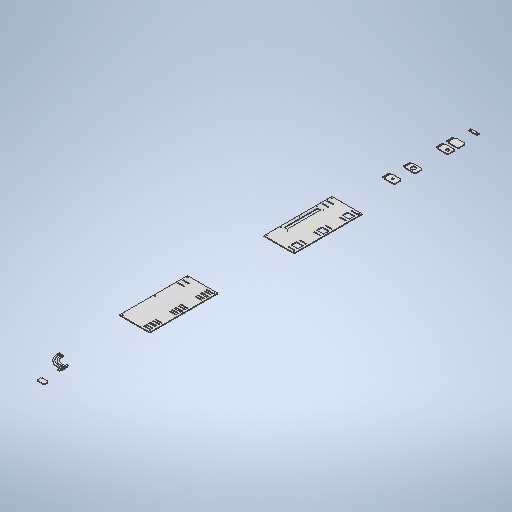
# Autodesk Inventor part: RAW_CHASSIS
Saved by Autodesk Inventor 2025 (Build 290162000, 162)
## iProperties
Created: 2024-11-01
Part Number: RAW_CHASSIS
Material: Generic
Document SubType Name: Modeling
Designer: Student
Density: 1 g/cm^3
Appearance: Default
Author: Student
Autodesk Inventor part; units mm, degrees
ref_plane "YZ Plane" through (0, 0, 0) normal (1, 0, 0) x (0, 1, 0)
ref_plane "XZ Plane" through (0, 0, 0) normal (0, 1, 0) x (-1, 0, 0)
ref_plane "XY Plane" through (0, 0, 0) normal (0, 0, 1) x (1, 0, 0)
sketch "Sketch1" plane through (0, 0, 0) normal (0, 1, 0) x (-1, 0, 0)
  point P0 (0, 0)
sketch "Sketch2" plane through (0, 0, 0) normal (0, 1, 0) x (-1, 0, 0)
  line L0 (-100, 225) -> (100, 225)
  line L1 (100, 225) -> (100, -225)
  line L2 (100, -225) -> (-100, -225)
  line L3 (-100, -225) -> (-100, 225)
  line L4 (-85, -35) -> (-45, -35)
  line L5 (-45, -35) -> (-45, -40)
  line L6 (-45, -40) -> (-85, -40)
  line L7 (-85, -40) -> (-85, -35)
  line L8 (-85, -35) -> (-45, -40) construction
  line L9 (-45, -35) -> (-85, -40) construction
  line L10 (-85, 35) -> (-45, 35)
  line L11 (-45, 35) -> (-45, 40)
  line L12 (-45, 40) -> (-85, 40)
  line L13 (-85, 40) -> (-85, 35)
  line L14 (-87.5, 188) -> (-42.5, 188)
  line L15 (-42.5, 188) -> (-42.5, 152)
  line L16 (-42.5, 152) -> (-87.5, 152)
  line L17 (-87.5, 152) -> (-87.5, 188)
  line L18 (-87.5, 188) -> (-42.5, 152) construction
  line L19 (-42.5, 188) -> (-87.5, 152) construction
  line L20 (-87.5, -188) -> (-42.5, -188)
  line L21 (-42.5, -188) -> (-42.5, -152)
  line L22 (-42.5, -152) -> (-87.5, -152)
  line L23 (-87.5, -152) -> (-87.5, -188)
  line L24 (-87.5, -188) -> (-42.5, -152) construction
  line L25 (-42.5, -188) -> (-87.5, -152) construction
  line L26 (-87.5, 18) -> (-42.5, 18)
  line L27 (-42.5, 18) -> (-42.5, -18)
  line L28 (-42.5, -18) -> (-87.5, -18)
  line L29 (-87.5, -18) -> (-87.5, 18)
  line L30 (-87.5, 18) -> (-42.5, -18) construction
  line L31 (-42.5, 18) -> (-87.5, -18) construction
  line L32 (100, 0) -> (70, 0)
  circle A0 centre (91, 120) radius 3
  circle A1 centre (49, 120) radius 3
  circle A2 centre (91, -120) radius 3
  circle A3 centre (49, -120) radius 3
  line L33 (50, -150) -> (90, -150)
  line L34 (90, -150) -> (90, -155)
  line L35 (90, -155) -> (50, -155)
  line L36 (50, -155) -> (50, -150)
  line L37 (50, -150) -> (90, -155) construction
  line L38 (90, -150) -> (50, -155) construction
  line L39 (50, -182) -> (90, -182)
  line L40 (90, -182) -> (90, -187)
  line L41 (90, -187) -> (50, -187)
  line L42 (50, -187) -> (50, -182)
  line L43 (50, -182) -> (90, -187) construction
  line L44 (90, -182) -> (50, -187) construction
  line L45 (60, 110) -> (80, 110)
  line L46 (80, 110) -> (80, -110)
  line L47 (80, -110) -> (60, -110)
  line L48 (60, -110) -> (60, 110)
  line L49 (60, 110) -> (80, -110) construction
  line L50 (80, 110) -> (60, -110) construction
  line L51 (100, 225) -> (80, 225)
  circle A4 centre (90, 215) radius 3
  circle A5 centre (90, -215) radius 3
  circle A6 centre (90, 0) radius 3
  circle A7 centre (-90, 215) radius 3
  circle A8 centre (-90, -215) radius 3
  circle A9 centre (-94, 0) radius 3
  line L52 (-76.0906, 1157.7188) -> (123.9094, 1157.7188)
  line L53 (123.9094, 1157.7188) -> (123.9094, 707.7188)
  line L54 (123.9094, 707.7188) -> (-76.0906, 707.7188)
  line L55 (-76.0906, 707.7188) -> (-76.0906, 1157.7188)
  line L56 (-61.0906, 1067.7188) -> (-21.0906, 1067.7188)
  line L57 (-21.0906, 1067.7188) -> (-21.0906, 1062.7188)
  line L58 (-21.0906, 1062.7188) -> (-61.0906, 1062.7188)
  line L59 (-61.0906, 1062.7188) -> (-61.0906, 1067.7188)
  line L60 (-61.0906, 1067.7188) -> (-21.0906, 1062.7188) construction
  line L61 (-21.0906, 1067.7188) -> (-61.0906, 1062.7188) construction
  line L62 (-61.0906, 897.7188) -> (-21.0906, 897.7188)
  line L63 (-21.0906, 897.7188) -> (-21.0906, 892.7188)
  line L64 (-21.0906, 892.7188) -> (-61.0906, 892.7188)
  line L65 (-61.0906, 892.7188) -> (-61.0906, 897.7188)
  line L66 (-61.0906, 897.7188) -> (-21.0906, 892.7188) construction
  line L67 (-21.0906, 897.7188) -> (-61.0906, 892.7188) construction
  line L68 (73.9094, 782.7188) -> (113.9094, 782.7188)
  line L69 (113.9094, 782.7188) -> (113.9094, 777.7188)
  line L70 (113.9094, 777.7188) -> (73.9094, 777.7188)
  line L71 (73.9094, 777.7188) -> (73.9094, 782.7188)
  line L72 (73.9094, 782.7188) -> (113.9094, 777.7188) construction
  line L73 (113.9094, 782.7188) -> (73.9094, 777.7188) construction
  line L74 (73.9094, 750.7188) -> (113.9094, 750.7188)
  line L75 (113.9094, 750.7188) -> (113.9094, 745.7188)
  line L76 (113.9094, 745.7188) -> (73.9094, 745.7188)
  line L77 (73.9094, 745.7188) -> (73.9094, 750.7188)
  line L78 (73.9094, 750.7188) -> (113.9094, 745.7188) construction
  line L79 (113.9094, 750.7188) -> (73.9094, 745.7188) construction
  line L80 (123.9094, 1157.7188) -> (103.9094, 1157.7188)
  circle A10 centre (113.9094, 1147.7188) radius 3
  circle A11 centre (113.9094, 717.7188) radius 3
  circle A12 centre (113.9094, 932.7188) radius 3
  circle A13 centre (-66.0906, 1147.7188) radius 3
  circle A14 centre (-66.0906, 717.7188) radius 3
  circle A15 centre (-70.0906, 932.7188) radius 3
  line L81 (-61.0906, 1096.7188) -> (-21.0906, 1096.7188)
  line L82 (-21.0906, 1096.7188) -> (-21.0906, 1108.7188)
  line L83 (-21.0906, 1108.7188) -> (-61.0906, 1108.7188)
  line L84 (-61.0906, 1108.7188) -> (-61.0906, 1096.7188)
  line L85 (-61.0906, 1096.7188) -> (-21.0906, 1108.7188) construction
  line L86 (-21.0906, 1096.7188) -> (-61.0906, 1108.7188) construction
  line L87 (-61.0906, 938.7188) -> (-21.0906, 938.7188)
  line L88 (-21.0906, 938.7188) -> (-21.0906, 926.7188)
  line L89 (-21.0906, 926.7188) -> (-61.0906, 926.7188)
  line L90 (-61.0906, 926.7188) -> (-61.0906, 938.7188)
  line L91 (-61.0906, 938.7188) -> (-21.0906, 926.7188) construction
  line L92 (-21.0906, 938.7188) -> (-61.0906, 926.7188) construction
  line L93 (-61.0906, 768.7188) -> (-21.0906, 768.7188)
  line L94 (-21.0906, 768.7188) -> (-21.0906, 756.7188)
  line L95 (-21.0906, 756.7188) -> (-61.0906, 756.7188)
  line L96 (-61.0906, 756.7188) -> (-61.0906, 768.7188)
  line L97 (-61.0906, 768.7188) -> (-21.0906, 756.7188) construction
  line L98 (-21.0906, 768.7188) -> (-61.0906, 756.7188) construction
  line L99 (-30, -502.9138) -> (30, -502.9138)
  line L100 (30, -552.9138) -> (-30, -552.9138)
  line L101 (-35, -547.9138) -> (-35, -507.9138)
  line L102 (-30, -507.9138) -> (30, -547.9138) construction
  line L103 (30, -507.9138) -> (-30, -547.9138) construction
  line L104 (30, -507.9138) -> (35, -507.9138)
  line L105 (30, -507.9138) -> (30, -502.9138)
  line L106 (30, -547.9138) -> (33, -547.9138)
  line L107 (-30, -507.9138) -> (-30, -502.9138)
  line L108 (-30, -507.9138) -> (-35, -507.9138)
  line L109 (-30, -547.9138) -> (-35, -547.9138)
  line L110 (-30, -547.9138) -> (-30, -552.9138)
  line L111 (30, -547.9138) -> (30, -552.9138)
  line L112 (30, -507.9138) -> (35, -507.9138)
  line L113 (35, -507.9138) -> (45, -507.9138)
  line L114 (45, -507.9138) -> (45, -547.9138)
  line L115 (45, -547.9138) -> (33, -547.9138)
  line L116 (35, -512.9138) -> (40, -512.9138)
  line L117 (40, -512.9138) -> (40, -542.9138)
  line L118 (40, -542.9138) -> (35, -542.9138)
  line L119 (35, -542.9138) -> (35, -512.9138)
  line L120 (35, -512.9138) -> (40, -542.9138) construction
  line L121 (40, -512.9138) -> (35, -542.9138) construction
  line L122 (-37.1604, -633.526) -> (22.8396, -633.526)
  line L123 (22.8396, -683.526) -> (-37.1604, -683.526)
  line L124 (-42.1604, -678.526) -> (-42.1604, -638.526)
  line L125 (-37.1604, -638.526) -> (22.8396, -678.526) construction
  line L126 (22.8396, -638.526) -> (-37.1604, -678.526) construction
  line L127 (22.8396, -638.526) -> (27.8396, -638.526)
  line L128 (22.8396, -638.526) -> (22.8396, -633.526)
  line L129 (22.8396, -678.526) -> (25.8396, -678.526)
  line L130 (-37.1604, -638.526) -> (-37.1604, -633.526)
  line L131 (-37.1604, -638.526) -> (-42.1604, -638.526)
  line L132 (-37.1604, -678.526) -> (-42.1604, -678.526)
  line L133 (-37.1604, -678.526) -> (-37.1604, -683.526)
  line L134 (22.8396, -678.526) -> (22.8396, -683.526)
  line L135 (22.8396, -638.526) -> (27.8396, -638.526)
  line L136 (27.8396, -638.526) -> (37.8396, -638.526)
  line L137 (37.8396, -638.526) -> (37.8396, -678.526)
  line L138 (37.8396, -678.526) -> (25.8396, -678.526)
  line L139 (27.8396, -643.526) -> (32.8396, -643.526)
  line L140 (32.8396, -643.526) -> (32.8396, -673.526)
  line L141 (32.8396, -673.526) -> (27.8396, -673.526)
  line L142 (27.8396, -673.526) -> (27.8396, -643.526)
  line L143 (27.8396, -643.526) -> (32.8396, -673.526) construction
  line L144 (32.8396, -643.526) -> (27.8396, -673.526) construction
  line L145 (-35.8287, -851.4704) -> (24.1713, -851.4704)
  line L146 (24.1713, -901.4704) -> (-35.8287, -901.4704)
  line L147 (-40.8287, -896.4704) -> (-40.8287, -856.4704)
  line L148 (-35.8287, -856.4704) -> (24.1713, -896.4704) construction
  line L149 (24.1713, -856.4704) -> (-35.8287, -896.4704) construction
  line L150 (24.1713, -856.4704) -> (29.1713, -856.4704)
  line L151 (24.1713, -856.4704) -> (24.1713, -851.4704)
  line L152 (24.1713, -896.4704) -> (27.1713, -896.4704)
  line L153 (-35.8287, -856.4704) -> (-35.8287, -851.4704)
  line L154 (-35.8287, -856.4704) -> (-40.8287, -856.4704)
  line L155 (-35.8287, -896.4704) -> (-40.8287, -896.4704)
  line L156 (-35.8287, -896.4704) -> (-35.8287, -901.4704)
  line L157 (24.1713, -896.4704) -> (24.1713, -901.4704)
  line L158 (24.1713, -856.4704) -> (29.1713, -856.4704)
  line L159 (29.1713, -856.4704) -> (39.1713, -856.4704)
  line L160 (39.1713, -856.4704) -> (39.1713, -896.4704)
  line L161 (39.1713, -896.4704) -> (27.1713, -896.4704)
  line L162 (29.1713, -861.4704) -> (34.1713, -861.4704)
  line L163 (34.1713, -861.4704) -> (34.1713, -891.4704)
  line L164 (34.1713, -891.4704) -> (29.1713, -891.4704)
  line L165 (29.1713, -891.4704) -> (29.1713, -861.4704)
  line L166 (29.1713, -861.4704) -> (34.1713, -891.4704) construction
  line L167 (34.1713, -861.4704) -> (29.1713, -891.4704) construction
  line L168 (-35.8287, -921.1593) -> (24.1713, -921.1593)
  line L169 (24.1713, -971.1593) -> (-35.8287, -971.1593)
  line L170 (-40.8287, -966.1593) -> (-40.8287, -926.1593)
  line L171 (-35.8287, -926.1593) -> (24.1713, -966.1593) construction
  line L172 (24.1713, -926.1593) -> (-35.8287, -966.1593) construction
  line L173 (24.1713, -926.1593) -> (29.1713, -926.1593)
  line L174 (24.1713, -926.1593) -> (24.1713, -921.1593)
  line L175 (24.1713, -966.1593) -> (27.1713, -966.1593)
  line L176 (-35.8287, -926.1593) -> (-35.8287, -921.1593)
  line L177 (-35.8287, -926.1593) -> (-40.8287, -926.1593)
  line L178 (-35.8287, -966.1593) -> (-40.8287, -966.1593)
  line L179 (-35.8287, -966.1593) -> (-35.8287, -971.1593)
  line L180 (24.1713, -966.1593) -> (24.1713, -971.1593)
  line L181 (24.1713, -926.1593) -> (29.1713, -926.1593)
  line L182 (29.1713, -926.1593) -> (39.1713, -926.1593)
  line L183 (39.1713, -926.1593) -> (39.1713, -966.1593)
  line L184 (39.1713, -966.1593) -> (27.1713, -966.1593)
  line L185 (29.1713, -931.1593) -> (34.1713, -931.1593)
  line L186 (34.1713, -931.1593) -> (34.1713, -961.1593)
  line L187 (34.1713, -961.1593) -> (29.1713, -961.1593)
  line L188 (29.1713, -961.1593) -> (29.1713, -931.1593)
  line L189 (29.1713, -931.1593) -> (34.1713, -961.1593) construction
  line L190 (34.1713, -931.1593) -> (29.1713, -961.1593) construction
  circle A16 centre (0, -527.9138) radius 7
  circle A17 centre (-7.1604, -658.526) radius 16.5
  line L191 (-61.0906, 1142.7188) -> (-21.0906, 1142.7188)
  line L192 (-21.0906, 1142.7188) -> (-21.0906, 1137.7188)
  line L193 (-21.0906, 1137.7188) -> (-61.0906, 1137.7188)
  line L194 (-61.0906, 1137.7188) -> (-61.0906, 1142.7188)
  line L195 (-61.0906, 1142.7188) -> (-21.0906, 1137.7188) construction
  line L196 (-21.0906, 1142.7188) -> (-61.0906, 1137.7188) construction
  line L197 (-61.0906, 1082.7188) -> (-21.0906, 1082.7188)
  line L198 (-21.0906, 1082.7188) -> (-21.0906, 1077.7188)
  line L199 (-21.0906, 1077.7188) -> (-61.0906, 1077.7188)
  line L200 (-61.0906, 1077.7188) -> (-61.0906, 1082.7188)
  line L201 (-61.0906, 1082.7188) -> (-21.0906, 1077.7188) construction
  line L202 (-21.0906, 1082.7188) -> (-61.0906, 1077.7188) construction
  line L203 (-61.0906, 1122.7188) -> (-21.0906, 1122.7188)
  line L204 (-21.0906, 1122.7188) -> (-21.0906, 1127.7188)
  line L205 (-21.0906, 1127.7188) -> (-61.0906, 1127.7188)
  line L206 (-61.0906, 1127.7188) -> (-61.0906, 1122.7188)
  line L207 (-61.0906, 912.7188) -> (-21.0906, 912.7188)
  line L208 (-21.0906, 912.7188) -> (-21.0906, 907.7188)
  line L209 (-21.0906, 907.7188) -> (-61.0906, 907.7188)
  line L210 (-61.0906, 907.7188) -> (-61.0906, 912.7188)
  line L211 (-61.0906, 912.7188) -> (-21.0906, 907.7188) construction
  line L212 (-21.0906, 912.7188) -> (-61.0906, 907.7188) construction
  line L213 (-41.0906, 932.7188) -> (-30, 932.7188)
  line L214 (-61.0906, 967.7188) -> (-21.0906, 967.7188)
  line L215 (-61.0906, 972.7188) -> (-61.0906, 967.7188)
  line L216 (-21.0906, 972.7188) -> (-61.0906, 972.7188)
  line L217 (-21.0906, 967.7188) -> (-21.0906, 972.7188)
  line L218 (-21.0906, 967.7188) -> (-61.0906, 972.7188) construction
  line L219 (-61.0906, 967.7188) -> (-21.0906, 972.7188) construction
  line L220 (-61.0906, 952.7188) -> (-21.0906, 952.7188)
  line L221 (-21.0906, 952.7188) -> (-21.0906, 957.7188)
  line L222 (-21.0906, 957.7188) -> (-61.0906, 957.7188)
  line L223 (-61.0906, 957.7188) -> (-61.0906, 952.7188)
  line L224 (-61.0906, 952.7188) -> (-21.0906, 957.7188) construction
  line L225 (-21.0906, 952.7188) -> (-61.0906, 957.7188) construction
  line L226 (-61.0906, 797.7188) -> (-21.0906, 797.7188)
  line L227 (-21.0906, 802.7188) -> (-61.0906, 802.7188)
  line L228 (-61.0906, 802.7188) -> (-61.0906, 797.7188)
  line L229 (-61.0906, 797.7188) -> (-21.0906, 802.7188) construction
  line L230 (-21.0906, 797.7188) -> (-61.0906, 802.7188) construction
  line L231 (-21.0906, 797.7188) -> (-21.0906, 802.7188)
  line L232 (-61.0906, 722.7188) -> (-21.0906, 722.7188)
  line L233 (-21.0906, 722.7188) -> (-21.0906, 727.7188)
  line L234 (-21.0906, 727.7188) -> (-61.0906, 727.7188)
  line L235 (-61.0906, 727.7188) -> (-61.0906, 722.7188)
  line L236 (-61.0906, 722.7188) -> (-21.0906, 727.7188) construction
  line L237 (-21.0906, 722.7188) -> (-61.0906, 727.7188) construction
  line L238 (-61.0906, 782.7188) -> (-21.0906, 782.7188)
  line L239 (-21.0906, 782.7188) -> (-21.0906, 787.7188)
  line L240 (-21.0906, 787.7188) -> (-61.0906, 787.7188)
  line L241 (-61.0906, 787.7188) -> (-61.0906, 782.7188)
  line L242 (-61.0906, 782.7188) -> (-21.0906, 787.7188) construction
  line L243 (-21.0906, 782.7188) -> (-61.0906, 787.7188) construction
  line L244 (-61.0906, 742.7188) -> (-21.0906, 742.7188)
  line L245 (-21.0906, 742.7188) -> (-21.0906, 737.7188)
  line L246 (-21.0906, 737.7188) -> (-61.0906, 737.7188)
  line L247 (-61.0906, 737.7188) -> (-61.0906, 742.7188)
  line L248 (-85, 135) -> (-45, 135)
  line L249 (-45, 135) -> (-45, 130)
  line L250 (-45, 130) -> (-85, 130)
  line L251 (-85, 130) -> (-85, 135)
  line L252 (-85, 135) -> (-45, 130) construction
  line L253 (-45, 135) -> (-85, 130) construction
  line L254 (-85, 205) -> (-45, 205)
  line L255 (-45, 205) -> (-45, 210)
  line L256 (-45, 210) -> (-85, 210)
  line L257 (-85, 210) -> (-85, 205)
  line L258 (-85, 205) -> (-45, 210) construction
  line L259 (-45, 205) -> (-85, 210) construction
  line L260 (-85, -135) -> (-45, -135)
  line L261 (-45, -135) -> (-45, -130)
  line L262 (-45, -130) -> (-85, -130)
  line L263 (-85, -130) -> (-85, -135)
  line L264 (-85, -135) -> (-45, -130) construction
  line L265 (-45, -135) -> (-85, -130) construction
  line L266 (-45, -205) -> (-45, -210)
  line L267 (-45, -210) -> (-85, -210)
  line L268 (-45, -205) -> (-85, -210) construction
  line L269 (-85, -205) -> (-45, -210) construction
  line L270 (-85, -210) -> (-85, -205)
  line L271 (-85, -205) -> (-45, -205)
  line L272 (-28, -1058.998) -> (28, -1058.998)
  line L273 (28, -1058.998) -> (28, -1073.998)
  line L274 (28, -1073.998) -> (-28, -1073.998)
  line L275 (-28, -1073.998) -> (-28, -1058.998)
  line L276 (-28, -1058.998) -> (28, -1073.998) construction
  line L277 (28, -1058.998) -> (-28, -1073.998) construction
  circle A18 centre (21, -1066.498) radius 3
  circle A19 centre (-21, -1066.498) radius 3
  circle A20 centre (-15.8287, -876.4704) radius 11
  point P0 (0, 0)
  point P1 (23.9094, 932.7188)
  point P2 (-41.0906, 762.7188)
  point P3 (-5.8287, -946.1593)
  dimension "d0" = 200
  dimension "d1" = 450
  dimension "d16" = 30
  dimension "d21" = 6
  dimension "d23" = 40
  dimension "d24" = 5
  dimension "d29" = 220
  dimension "d32" = 6
  dimension "d33" = 6
  dimension "d36" = 200
  dimension "d37" = 450
  dimension "d40" = 40
  dimension "d41" = 5
  dimension "d43" = 6
  dimension "d44" = 6
  dimension "d46" = 12
  dimension "d47" = 40
  dimension "d51" = 60
  dimension "d61" = 60
  dimension "d62" = 60
  dimension "d63" = 60
  dimension "d64" = 14
  dimension "d70" = 5
  dimension "d72" = 5
  dimension "d75" = 40
  dimension "d76" = 5
  dimension "d79" = 40
  dimension "d80" = 5
  dimension "d82" = 56
  dimension "d83" = 15
  dimension "d85" = 6
  dimension "d88" = 36
  dimension "d89" = 45
  constraints: 556 end point, 51 perpendicular, 50 parallel, 39 horizontal, 27 symmetric about line, 21 centre point, 10 midpoint, 5 point on line, 2 coincident, 3 other
  measures "d0" distance of L1.end L2.end
  measures "d1" distance of L0.end L1.end
  measures "d16" distance of L32.start L32.end
  measures "d21" diameter of A0
  measures "d23" distance of L34.end L35.end
  measures "d24" distance of L33.end L34.end
  measures "d29" distance of L45.end L46.end
  measures "d32" diameter of A4
  measures "d33" diameter of A6
  measures "d36" distance of L53.end L55.start
  measures "d37" distance of L52.end L53.end
  measures "d40" distance of L70.start L71.start
  measures "d41" distance of L68.end L70.start
  measures "d43" diameter of A10
  measures "d44" diameter of A12
  measures "d46" distance of L82.end L81.end
  measures "d47" distance of L88.end L89.end
  measures "d51" distance of L102.end L103.end
  measures "d61" distance of L134.start L126.end
  measures "d62" distance of L157.start L149.end
  measures "d63" distance of L180.start L172.end
  measures "d64" diameter of A16
  measures "d70" distance of L191.end L192.end
  measures "d72" distance of L197.end L198.end
  measures "d75" distance of L208.end L209.end
  measures "d76" distance of L207.end L208.end
  measures "d79" distance of L249.end L250.end
  measures "d80" distance of L248.end L249.end
  measures "d82" distance of L273.end L274.end
  measures "d83" distance of L272.end L273.end
  measures "d85" diameter of A18
  measures "d88" distance of L16.end L14.start
  measures "d89" distance of L14.start L14.end
extrude "Extrusion1" add sketch "Sketch2" along normal blind 5
sketch "Sketch3" plane through (0, 0, 0) normal (0, 1, 0) x (-1, 0, 0)
  line L0 (0, 1665.8573) -> (5, 1665.8573)
  line L1 (5, 1625.8573) -> (0, 1625.8573)
  line L2 (0, 1625.8573) -> (0, 1665.8573)
  line L3 (5, 1625.8573) -> (5, 1615.8573)
  line L4 (5, 1615.8573) -> (15, 1615.8573)
  line L5 (15, 1675.8573) -> (5, 1675.8573)
  line L6 (5, 1660.8573) -> (10, 1660.8573)
  line L7 (10, 1660.8573) -> (10, 1630.8573)
  line L8 (10, 1630.8573) -> (5, 1630.8573)
  line L9 (5, 1630.8573) -> (5, 1660.8573)
  line L10 (5, 1660.8573) -> (10, 1630.8573) construction
  line L11 (10, 1660.8573) -> (5, 1630.8573) construction
  line L12 (5, 1675.8573) -> (5, 1665.8573)
  line L13 (15, 1660.8573) -> (35, 1660.8573)
  line L14 (15, 1630.8573) -> (35, 1630.8573)
  line L15 (15, 1651.3573) -> (35, 1651.3573)
  line L16 (15, 1640.3573) -> (35, 1640.3573)
  line L17 (15, 1615.8573) -> (15, 1630.8573)
  line L18 (15, 1675.8573) -> (15, 1660.8573)
  line L19 (85, 1590.3573) -> (96, 1590.3573)
  arc A0 (96, 1590.3573) -> (35, 1651.3573) centre (35, 1590.3573) ccw
  arc A1 (85, 1590.3573) -> (35, 1640.3573) centre (35, 1590.3573) ccw
  line L20 (15, 1660.8573) -> (35, 1660.8573)
  arc A2 (105.5, 1590.3573) -> (35, 1660.8573) centre (35, 1590.3573) ccw
  arc A3 (75.5, 1590.3573) -> (35, 1630.8573) centre (35, 1590.3573) ccw
  line L21 (35, 1630.8573) -> (15, 1630.8573)
  line L22 (105.5, 1590.3573) -> (105.5, 1575.3573)
  line L23 (75.5, 1590.3573) -> (75.5, 1575.3573)
  line L24 (75.5, 1575.3573) -> (104.857, 1575.3573)
  line L25 (105.5, 1575.3573) -> (104.857, 1575.3573)
  line L26 (80.5, 1585.3573) -> (100.5, 1585.3573)
  line L27 (100.5, 1585.3573) -> (100.5, 1580.3573)
  line L28 (100.5, 1580.3573) -> (80.5, 1580.3573)
  line L29 (80.5, 1580.3573) -> (80.5, 1585.3573)
  line L30 (80.5, 1585.3573) -> (100.5, 1580.3573) construction
  line L31 (100.5, 1585.3573) -> (80.5, 1580.3573) construction
  line L32 (15, 1651.3573) -> (15, 1640.3573)
  line L33 (-19, 1805.4917) -> (19, 1805.4917)
  line L34 (19, 1775.4917) -> (-19, 1775.4917)
  line L35 (-19, 1805.4917) -> (19, 1775.4917) construction
  line L36 (19, 1805.4917) -> (-19, 1775.4917) construction
  line L37 (19, 1805.4917) -> (19, 1800.4917)
  line L38 (19, 1800.4917) -> (24, 1800.4917)
  line L39 (24, 1800.4917) -> (24, 1780.4917)
  line L40 (24, 1780.4917) -> (19, 1780.4917)
  line L41 (19, 1775.4917) -> (19, 1780.4917)
  line L42 (-19, 1800.4917) -> (-24, 1800.4917)
  line L43 (-24, 1800.4917) -> (-24, 1780.4917)
  line L44 (-24, 1780.4917) -> (-19, 1780.4917)
  line L45 (-19, 1775.4917) -> (-19, 1780.4917)
  line L46 (-19, 1800.4917) -> (-19, 1805.4917)
  point P0 (0, 0)
  point P1 (90.5, 1582.8573)
  dimension "d92" = 5
  dimension "d93" = 40
  dimension "d94" = 10
  dimension "d95" = 10
  dimension "d96" = 60
  dimension "d99" = 30
  dimension "d100" = 20
  dimension "d101" = 20
  dimension "d102" = 9.5
  dimension "d103" = 9.5
  dimension "d107" = 61
  dimension "d108" = 50
  dimension "d109" = 9.5
  dimension "d113" = 38
  dimension "d114" = 30
  dimension "d115" = 5
  dimension "d116" = 5
  dimension "d117" = 20
  constraints: 94 end point, 8 point on circle, 7 horizontal, 7 parallel, 7 vertical, 5 perpendicular, 4 centre point, 2 collinear, 2 midpoint
  measures "d92" distance of L1.start L1.end
  measures "d93" distance of L0.end L1.start
  measures "d94" distance of L1.start L3.end
  measures "d95" distance of L5.end L5.start
  measures "d96" distance of L5.start L4.end
  measures "d99" distance of L6.end L7.end
  measures "d100" distance of L13.start L13.end
  measures "d101" distance of L14.start L14.end
  measures "d102" distance of L13.start L15.start
  measures "d103" distance of L14.start L16.start
  measures "d107" radius of A0
  measures "d108" radius of A1
  measures "d109" radial gap between concentric circles of A0 A2
  measures "d113" distance of L34.start L34.end
  measures "d114" distance of L33.end L34.start
  measures "d115" distance of L33.end L37.end
  measures "d116" distance of L37.end L38.end
  measures "d117" distance of L38.end L39.end
extrude "Extrusion2" add sketch "Sketch3" along normal blind 5
body "Solid1"
